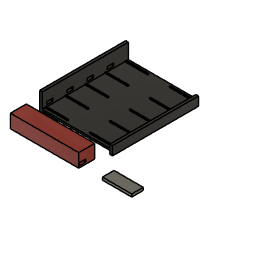
paccoBatterie v2 (Autodesk Fusion 360 archive; units mm, degrees)
design "paccoBatterie"
part number: Configurazione 1
Autodesk Fusion 360 part; units mm, degrees
sketch "Schizzo1" plane through (0, 0, 0) normal (0, 0, 1) x (1, 0, 0)
  line L0 (0, 0) -> (-77, 0)
  line L1 (-77, 0) -> (-77, 18)
  line L2 (-77, 18) -> (0, 18)
  line L3 (0, 18) -> (0, 0)
  line L4 (25, 1.7) -> (58, 1.7)
  line L5 (58, 1.7) -> (58, 14.7)
  line L6 (58, 14.7) -> (25, 14.7)
  line L7 (25, 14.7) -> (25, 1.7)
  dimension "d1" = 77
  dimension "d2" = 18
  dimension "d3" = 33
  dimension "d4" = 13
  constraint coincident L0.start L3.end
  constraint horizontal L0
  constraint perpendicular L0 L1
  constraint perpendicular L1 L2
  constraint perpendicular L0 L3
  constraint perpendicular L3 L4
  constraint perpendicular L4 L5
  constraint perpendicular L5 L6
  constraint perpendicular L4 L7
  measures "d1" distance of L0.start L0.end
  measures "d2" distance of L0.end L1.end
  measures "d3" distance of L4.start L4.end
  measures "d4" distance of L4.end L5.end
extrude "Estrusione1" add sketch "Schizzo1" along normal blind 15.2 contours L0 L1 L2 L3 makes body 1
extrude "Estrusione2" add sketch "Schizzo1" along normal blind 3 separate body contours L4 L5 L6 L7 makes body 2
sketch "Schizzo2" plane through (0, 0, 0) normal (0, 0, 1) x (1, 0, 0)
  line L0 (0, 35) -> (-76, 35)
  line L1 (-76, 35) -> (-76, 132)
  line L2 (-76, 132) -> (0, 132)
  line L3 (0, 35) -> (3, 35)
  line L4 (3, 35) -> (3, 132)
  line L5 (3, 132) -> (0, 132)
  line L6 (0, 132) -> (0, 35)
  line L7 (-76, 35) -> (-79, 35)
  line L8 (-79, 35) -> (-79, 132)
  line L9 (-79, 132) -> (-76, 132)
  line L10 (-76, 132) -> (-76, 35)
  dimension "d9" = 76
  dimension "d10" = 97
  dimension "d12" = 3
  dimension "d13" = 3
  constraint horizontal L0
  constraint vertical L1
  constraint horizontal L2
  constraint horizontal L3
  constraint vertical L4
  constraint horizontal L5
  constraint vertical L6
  constraint horizontal L7
  constraint vertical L8
  constraint horizontal L9
  constraint vertical L10
  measures "d9" distance of L0.start L0.end
  measures "d10" distance of L0.start L2.end
  measures "d12" distance of L0.start L3.end
  measures "d13" distance of L0.end L7.end
extrude "Estrusione3" add sketch "Schizzo2" along normal blind 2 separate body contours L0 L1 L2 L6 L10 makes body 3
extrude "Estrusione4" add sketch "Schizzo2" along normal blind 19 contours L3 L4 L5 L6 | L1 L7 L8 L9 L10 bodies 3
extrude "Estrusione6" add sketch "Schizzo2" against normal blind 17 contours L3 L4 L5 L6 | L1 L7 L8 L9 L10 bodies 3
sketch "Schizzo3" plane through (0, 0, 2) normal (0, 0, 1) x (-1, 0, 0)
  line L0 (0, -132) -> (76, -132)
  line L1 (76, -132) -> (76, -35)
  line L2 (76, -35) -> (0, -35)
  line L3 (0, -35) -> (0, -132)
  line L4 (0, -38) -> (26, -38)
  line L5 (26, -38) -> (26, -39)
  line L6 (26, -39) -> (0, -39)
  line L7 (0, -39) -> (0, -38)
  line L8 (76, -38) -> (50, -38)
  line L9 (50, -38) -> (50, -39)
  line L10 (50, -39) -> (76, -39)
  line L11 (76, -39) -> (76, -38)
  dimension "d45" = 26
  dimension "d46" = 1
  dimension "d47" = 26
  dimension "d48" = 1
  dimension "d49" = 3
  dimension "d50" = 3
  constraint horizontal L4
  constraint vertical L5
  constraint horizontal L6
  constraint vertical L7
  constraint coincident L3 L4.start
  constraint horizontal L8
  constraint vertical L9
  constraint horizontal L10
  constraint vertical L11
  constraint coincident L1 L8.start
  measures "d45" distance of L4.start L4.end
  measures "d46" distance of L4.start L6.end
  measures "d47" distance of L8.start L8.end
  measures "d48" distance of L8.start L10.end
  measures "d49" distance of L2 L8
  measures "d50" distance of L2 L4
extrude "Estrusione8" add sketch "Schizzo3" along normal blind 1 contours L3 L4 L5 L6 L7 | L1 L8 L9 L10 L11 bodies 3
pattern_linear "Serie R2" count 5 spacing 22.5 along (0, 1, 0) of "Estrusione8"
sketch "Schizzo4" plane through (0, 0, 0) normal (0, 0, -1) x (1, 0, 0)
  line L0 (-76, -35) -> (-76, -132)
  line L1 (-76, -132) -> (0, -132)
  line L2 (0, -132) -> (0, -35)
  line L3 (0, -35) -> (-76, -35)
  line L4 (-76, -38) -> (-50, -38)
  line L5 (-50, -38) -> (-50, -39)
  line L6 (-50, -39) -> (-76, -39)
  line L7 (-76, -39) -> (-76, -38)
  line L8 (0, -38) -> (-26, -38)
  line L9 (-26, -38) -> (-26, -39)
  line L10 (-26, -39) -> (0, -39)
  line L11 (0, -39) -> (0, -38)
  line L12 (0, -35) -> (-76, -35)
  dimension "d57" = 1
  dimension "d58" = 26
  dimension "d59" = 1
  dimension "d60" = 3
  dimension "d61" = 3
  constraint horizontal L4
  constraint vertical L5
  constraint horizontal L6
  constraint vertical L7
  constraint coincident L0 L4.start
  constraint horizontal L8
  constraint vertical L9
  constraint horizontal L10
  constraint vertical L11
  constraint coincident L2 L8.start
  measures "d57" distance of L4.start L6.end
  measures "d58" distance of L8.start L8.end
  measures "d59" distance of L8.start L10.end
  measures "d60" distance of L8 L12
  measures "d61" distance of L4 L12
extrude "Estrusione9" add sketch "Schizzo4" along normal blind 1 contours L0 L4 L5 L6 L7 | L2 L8 L9 L10 L11 bodies 3
pattern_linear "Serie R3" count 5 spacing 22.5 along (0, 1, 0) of "Estrusione9"
sketch "Schizzo5" plane through (-77, 0, 0) normal (-1, 0, 0) x (0, -1, 0)
  line L0 (-18, 0) -> (0, 0)
  line L1 (0, 0) -> (0, 15.2)
  line L2 (0, 15.2) -> (-18, 15.2)
  line L3 (-18, 15.2) -> (-18, 0)
  line L4 (-1, 2) -> (-8, 2)
  line L5 (-8, 2) -> (-8, 5)
  line L6 (-8, 5) -> (-1, 5)
  line L7 (-1, 5) -> (-1, 2)
  dimension "d68" = 7
  dimension "d69" = 3
  dimension "d70" = 2
  dimension "d71" = 1
  constraint horizontal L4
  constraint vertical L5
  constraint horizontal L6
  constraint vertical L7
  measures "d68" distance of L4.start L4.end
  measures "d69" distance of L4.start L6.end
  measures "d70" distance of L0 L4
  measures "d71" distance of L1 L7
extrude "Estrusione10" cut sketch "Schizzo5" against normal blind 80 contours L4 L5 L6 L7 bodies 1
sketch "Schizzo7" plane through (-76, 0, 0) normal (1, 0, 0) x (0, 1, 0)
  line L0 (128, 2) -> (128, 3)
  line L1 (128, 3) -> (129, 3)
  line L2 (129, 3) -> (129, 2)
  line L3 (129, 2) -> (132, 2)
  line L4 (132, 2) -> (132, 19)
  line L5 (132, 19) -> (35, 19)
  line L6 (35, 19) -> (35, 2)
  line L7 (35, 2) -> (38, 2)
  line L8 (38, 2) -> (38, 3)
  line L9 (38, 3) -> (39, 3)
  line L10 (39, 3) -> (39, 2)
  line L11 (39, 2) -> (60.5, 2)
  line L12 (60.5, 2) -> (60.5, 3)
  line L13 (60.5, 3) -> (61.5, 3)
  line L14 (61.5, 3) -> (61.5, 2)
  line L15 (61.5, 2) -> (83, 2)
  line L16 (83, 2) -> (83, 3)
  line L17 (83, 3) -> (84, 3)
  line L18 (84, 3) -> (84, 2)
  line L19 (84, 2) -> (105.5, 2)
  line L20 (105.5, 2) -> (105.5, 3)
  line L21 (105.5, 3) -> (106.5, 3)
  line L22 (106.5, 3) -> (106.5, 2)
  line L23 (106.5, 2) -> (128, 2)
  line L24 (40, 7) -> (47, 7)
  line L25 (47, 7) -> (47, 4)
  line L26 (47, 4) -> (40, 4)
  line L27 (40, 4) -> (40, 7)
  dimension "d79" = 7
  dimension "d80" = 3
  dimension "d81" = 2
  dimension "d82" = 5
  constraint horizontal L24
  constraint vertical L25
  constraint horizontal L26
  constraint vertical L27
  measures "d79" distance of L24.start L24.end
  measures "d80" distance of L24.start L26.end
  measures "d81" distance of L11 L26
  measures "d82" distance of L6 L26.end
extrude "Estrusione11" cut sketch "Schizzo7" against normal blind 3 contours L24 L25 L26 L27 bodies 3
pattern_linear "Serie R4" count 2 spacing 9 along (0, 0, -1) count 4 spacing 22.75 along (0, 1, 0) of "Estrusione11"
extrude "Estrusione12" cut 1 faces at (1, 67.3333, 19) along direction (0, 0, -1) blind 13 on bodies 3 bodies 3
extrude "Estrusione13" cut 1 faces at (1, 67.3333, -17) along direction (0, 0, 1) blind 13 on bodies 3 bodies 3
equation "d9 = lunghezza"
equation "d10 = largezza"
equation "d12 = spessoreLato"
equation "d13 = spessoreLato"
equation "d14 = spessorePiano"
equation "d16 = altezza"
equation "d20 = altezzaNegativa"
equation "spessoreLato = 3 mm"
equation "spessorePiano = 2 mm"
equation "largezza = ( spessoreIncastro + largezzaBattreia ) * Nbatterie + 2 * margine"
equation "lunghezza = 76 mm"
equation "altezza = spessorePiano + 17 mm"
equation "altezzaNegativa = -( altezza - spessorePiano )"
equation "margine = 3 mm"
equation "largezzaBattreia = 21.75 mm"
equation "spessoreIncastro = 1 mm"
equation "Nbatterie = 4"
equation "d46 = spessoreIncastro"
equation "d48 = spessoreIncastro"
equation "d49 = margine"
equation "d50 = margine"
equation "d53 = Nbatterie + 1"
equation "d55 = ( largezzaBattreia + spessoreIncastro ) * Nbatterie - spessoreIncastro"
equation "d57 = spessoreIncastro"
equation "d59 = spessoreIncastro"
equation "d60 = margine"
equation "d61 = margine"
equation "d62 = spessoreIncastro"
equation "d64 = Nbatterie + 1"
equation "d66 = ( largezzaBattreia + spessoreIncastro ) * Nbatterie - spessoreIncastro"
equation "d82 = margine + spessoreIncastro + 1 mm"
equation "d83 = -spessoreLato"
equation "d86 = Nbatterie"
equation "d87 = -7 mm - spessorePiano"
equation "d88 = ( largezzaBattreia + spessoreIncastro ) * ( Nbatterie - 1 )"
equation "d95 = 0 mm - 13 mm"
